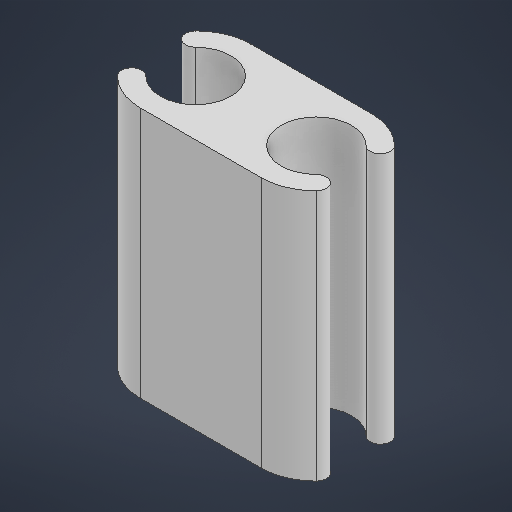
# Autodesk Inventor part: 카메라 고정 중단
Saved by Autodesk Inventor 2026.2 (Build 302298000, 298)
## iProperties
Created: 2025-11-20
Part Number: 카메라 고정 중단
Material: 일반
Document SubType Name: Modeling
Designer: PC
Density: 1 g/cm^3
Appearance: 기본값
Author: PC
Autodesk Inventor part; units mm, degrees
ref_plane "YZ Plane" through (0, 0, 0) normal (1, 0, 0) x (0, 1, 0)
ref_plane "XZ Plane" through (0, 0, 0) normal (0, 1, 0) x (-1, 0, 0)
ref_plane "XY Plane" through (0, 0, 0) normal (0, 0, 1) x (1, 0, 0)
sketch "스케치1" plane through (0, 0, 0) normal (0, 1, 0) x (-1, 0, 0)
  line L0 (0, -16.483) -> (0, 16.483) projected
  line L1 (31.8385, 0) -> (-30.0309, 0) projected
  arc A0 (16.9497, 4.9497) -> (16.9497, -4.9497) centre (12, 0) ccw
  line L2 (12, -11) -> (0, -11)
  line L3 (12, 11) -> (0, 11)
  line L4 (12, 0) -> (19.7782, -7.7782)
  line L5 (12, 0) -> (23, 0) construction
  arc A1 (19.7782, -7.7782) -> (16.9497, -4.9497) centre (18.364, -6.364) ccw
  arc A2 (16.9497, 4.9497) -> (19.7782, 7.7782) centre (18.364, 6.364) ccw
  arc A3 (12, -11) -> (19.7782, -7.7782) centre (12, 0) ccw
  arc A4 (19.7782, 7.7782) -> (12, 11) centre (12, 0) ccw
  arc A5 (-16.9497, -4.9497) -> (-16.9497, 4.9497) centre (-12, 0) ccw
  line L6 (-12, -11) -> (0, -11)
  arc A6 (-16.9497, -4.9497) -> (-19.7782, -7.7782) centre (-18.364, -6.364) ccw
  arc A7 (-19.7782, 7.7782) -> (-16.9497, 4.9497) centre (-18.364, 6.364) ccw
  arc A8 (-19.7782, -7.7782) -> (-12, -11) centre (-12, 0) ccw
  arc A9 (-12, 11) -> (-19.7782, 7.7782) centre (-12, 0) ccw
  line L7 (-12, 11) -> (0, 11)
  point P0 (0, 0)
  dimension "d0" = 14
  dimension "d1" = 12
  dimension "d3" = 45
  dimension "d4" = 11
  constraints: 20 point on circle, 12 end point, 12 symmetric about line, 10 centre point, 4 point on line, 3 tangent, 2 perpendicular, 1 equal length, 1 horizontal, 6 other
  measures "d0" diameter of A0
  measures "d1" distance of point (0, 0) L4.start
  measures "d3" angle of L4 L5
  measures "d4" radius of A3
extrude "돌출1" add sketch "스케치1" along normal blind 50 contours L6 A8 A6 A5 L1 L0 | L0 L1 A0 L4 A3 L2 | L1 A5 A7 A9 L7 L0 | L0 L3 A4 A2 A0 L1 | L4 A1
